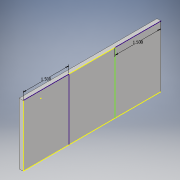
# Autodesk Inventor part: bottom near wheel 4.5x2
Saved by Autodesk Inventor 2017 (Build 210142000, 142)
## iProperties
Created: 2017-03-02
Part Number: bottom near wheel 4.5x2
Material: Generic
Document SubType Name: Modeling
Designer: Jess
Density: 1 g/cm^3
Appearance: Default
Author: Jess
Autodesk Inventor part; units mm, degrees
ref_plane "YZ Plane" through (0, 0, 0) normal (1, 0, 0) x (0, 1, 0)
ref_plane "XZ Plane" through (0, 0, 0) normal (0, 1, 0) x (-1, 0, 0)
ref_plane "XY Plane" through (0, 0, 0) normal (0, 0, 1) x (1, 0, 0)
sketch "Sketch1" plane through (0, 0, 0) normal (1, 0, 0) x (0, 1, 0)
  line L0 (5.846, 14.6477) -> (-44.954, 14.6477)
  line L1 (-44.954, 14.6477) -> (-44.954, -99.6523)
  line L2 (-44.954, -99.6523) -> (5.846, -99.6523)
  line L3 (5.846, -99.6523) -> (5.846, 14.6477)
  point P0 (0, 0)
  dimension "d0" = 50.8
  dimension "d1" = 114.3
  constraints: 8 end point, 2 parallel, 1 horizontal, 1 perpendicular
  measures "d0" distance of L2.end L1.end
  measures "d1" distance of L1.end L0.end
extrude "Extrusion1" add sketch "Sketch1" along normal blind 3.175
sketch "Sketch2" plane through (3.175, 0, 0) normal (1, 0, 0) x (0, 0, -1)
  line L0 (-14.6477, 5.846) -> (-14.6477, -44.954) projected
  line L1 (-14.6477, 5.846) -> (23.4523, 5.846)
  line L2 (99.6523, 5.846) -> (-14.6477, 5.846) projected
  line L3 (23.4523, 5.846) -> (23.4523, -44.954)
  line L4 (-14.6477, -44.954) -> (99.6523, -44.954) projected
  line L5 (99.6523, 5.846) -> (61.5523, 5.846)
  line L6 (61.5523, 5.846) -> (61.5523, -44.954)
  line L7 (61.5523, 5.846) -> (61.5523, -44.954)
  point P0 (0, 0)
  dimension "d4" = 38.1
  dimension "d5" = 38.1
  constraints: 10 end point, 4 point on line, 2 perpendicular, 1 collinear
  measures "d4" distance of L0.start L1.end
  measures "d5" distance of L5.start L5.end
body "Solid1"
